Autodesk Inventor part; units mm, degrees
(part 3 of 3)
sketch "Эскиз41" plane through (1.5, 0, 0) normal (1, 0, 0) x (0, 0, -1)
  circle A0 centre (383.6, 368.9) radius 1.625 projected
  circle A1 centre (-13.6, 369) radius 1.625 projected
  circle A2 centre (383.6, 1.1) radius 1.625 projected
  circle A3 centre (-13.6, 1.1) radius 1.625 projected
  circle A4 centre (379.0468, 185.0848) radius 1.625 projected
  circle A5 centre (-9.0468, 185.0848) radius 1.625 projected
  circle A6 centre (379, 228) radius 1.625 projected
  circle A7 centre (-9, 228) radius 1.625 projected
  circle A8 centre (316, 368) radius 1.625 projected
  circle A9 centre (299, 228) radius 1.625 projected
  circle A10 centre (54, 228) radius 1.625 projected
  circle A11 centre (71, 142) radius 1.625 projected
  circle A12 centre (71, 2.0002) radius 1.625 projected
  circle A13 centre (54, 2.0002) radius 1.625 projected
  circle A14 centre (71, 368) radius 1.625 projected
  circle A15 centre (71, 228) radius 1.625 projected
  circle A16 centre (316, 142) radius 1.625 projected
  circle A17 centre (316, 228) radius 1.625 projected
  circle A18 centre (183.175, 129.0059) radius 1.85 projected
  circle A19 centre (299, 368) radius 1.625 projected
  circle A20 centre (316, 2.0002) radius 1.625 projected
  circle A21 centre (54, 142) radius 1.625 projected
  circle A22 centre (54, 368) radius 1.625 projected
  circle A23 centre (299, 2.0002) radius 1.625 projected
  circle A24 centre (299, 142) radius 1.625 projected
  arc A25 (185, 193.309) -> (185, 192.7028) centre (183.175, 193.0059) ccw projected
  line L0 (185, 193.309) -> (185, 192.7028) projected
  line L1 (14.5, 247.5001) -> (35, 247.5001) projected
  arc A26 (38, 244.5001) -> (35, 247.5001) centre (35, 244.5001) ccw projected
  line L2 (38, 244.5001) -> (38, 185.5001) projected
  arc A27 (35, 182.5001) -> (38, 185.5001) centre (35, 185.5001) ccw projected
  line L3 (35, 182.5001) -> (14.5, 182.5001) projected
  arc A28 (11.5, 185.5001) -> (14.5, 182.5001) centre (14.5, 185.5001) ccw projected
  line L4 (11.5, 185.5001) -> (11.5, 244.5001) projected
  arc A29 (14.5, 247.5001) -> (11.5, 244.5001) centre (14.5, 244.5001) ccw projected
  line L5 (358.5, 244.5001) -> (358.5, 185.5001) projected
  arc A30 (355.5, 182.5001) -> (358.5, 185.5001) centre (355.5, 185.5001) ccw projected
  line L6 (355.5, 182.5001) -> (335, 182.5001) projected
  arc A31 (332, 185.5001) -> (335, 182.5001) centre (335, 185.5001) ccw projected
  line L7 (332, 185.5001) -> (332, 244.5001) projected
  arc A32 (335, 247.5001) -> (332, 244.5001) centre (335, 244.5001) ccw projected
  line L8 (335, 247.5001) -> (355.5, 247.5001) projected
  arc A33 (358.5, 244.5001) -> (355.5, 247.5001) centre (355.5, 244.5001) ccw projected
  line L9 (98.825, 226.3849) -> (98.825, 137.3849) projected
  arc A34 (95.825, 134.3849) -> (98.825, 137.3849) centre (95.825, 137.3849) ccw projected
  line L10 (95.825, 134.3849) -> (87.825, 134.3849) projected
  arc A35 (84.825, 137.3849) -> (87.825, 134.3849) centre (87.825, 137.3849) ccw projected
  line L11 (84.825, 137.3849) -> (84.825, 226.3849) projected
  arc A36 (87.825, 229.3849) -> (84.825, 226.3849) centre (87.825, 226.3849) ccw projected
  line L12 (87.825, 229.3849) -> (95.825, 229.3849) projected
  arc A37 (98.825, 226.3849) -> (95.825, 229.3849) centre (95.825, 226.3849) ccw projected
  circle A38 centre (124.375, 129.0059) radius 2 projected
  circle A39 centre (124.375, 193.0059) radius 2 projected
  circle A40 centre (217.25, 312.9941) radius 2.1 projected
  circle A41 centre (152.75, 57.0059) radius 2.1 projected
  circle A42 centre (152.75, 118.0059) radius 2.1 projected
  circle A43 centre (152.75, 312.9941) radius 2.1 projected
  circle A44 centre (217.25, 251.9941) radius 2.1 projected
  circle A45 centre (217.25, 57.0059) radius 2.1 projected
  circle A46 centre (217.25, 118.0059) radius 2.1 projected
  circle A47 centre (152.75, 251.9941) radius 2.1 projected
  line L13 (165, 44) -> (165, 8) projected
  arc A48 (162, 5) -> (165, 8) centre (162, 8) ccw projected
  line L14 (162, 5) -> (96, 5) projected
  arc A49 (93, 8) -> (96, 5) centre (96, 8) ccw projected
  line L15 (93, 8) -> (93, 44) projected
  arc A50 (96, 47) -> (93, 44) centre (96, 44) ccw projected
  line L16 (96, 47) -> (162, 47) projected
  arc A51 (165, 44) -> (162, 47) centre (162, 44) ccw projected
  circle A52 centre (319.1128, 165.0002) radius 2.1 projected
  circle A53 centre (287, 56.343) radius 2.1 projected
  circle A54 centre (50.8872, 165.0002) radius 2.1 projected
  circle A55 centre (173.9908, 56.343) radius 2.1 projected
  circle A56 centre (135.25, 60) radius 2.1 projected
  circle A57 centre (103, 60) radius 2.1 projected
  line L17 (226.25, 270.0041) -> (226.25, 298.657) projected
  arc A58 (228.25, 300.657) -> (226.25, 298.657) centre (228.25, 298.657) ccw projected
  line L18 (228.25, 300.657) -> (268.3252, 300.657) projected
  arc A59 (269.4885, 297.03) -> (268.3252, 300.657) centre (268.3252, 298.657) ccw projected
  line L19 (269.4885, 297.03) -> (229.4132, 268.3772) projected
  arc A60 (226.25, 270.0041) -> (229.4132, 268.3772) centre (228.25, 270.0041) ccw projected
  arc A61 (235.9248, 170.343) -> (234.7615, 166.7161) centre (235.9248, 168.343) ccw projected
  line L20 (235.9248, 170.343) -> (276, 170.343) projected
  arc A62 (278, 168.343) -> (276, 170.343) centre (276, 168.343) ccw projected
  line L21 (278, 168.343) -> (278, 139.6902) projected
  arc A63 (274.8368, 138.0633) -> (278, 139.6902) centre (276, 139.6902) ccw projected
  line L22 (274.8368, 138.0633) -> (234.7615, 166.7161) projected
  arc A64 (94, 106.343) -> (92, 104.343) centre (94, 104.343) ccw projected
  line L23 (94, 106.343) -> (134.0752, 106.343) projected
  arc A65 (135.2385, 102.7161) -> (134.0752, 106.343) centre (134.0752, 104.343) ccw projected
  line L24 (135.2385, 102.7161) -> (95.1632, 74.0633) projected
  arc A66 (92, 75.6902) -> (95.1632, 74.0633) centre (94, 75.6902) ccw projected
  line L25 (92, 75.6902) -> (92, 104.343) projected
  arc A67 (92, 265.657) -> (94, 263.657) centre (94, 265.657) ccw projected
  line L26 (92, 265.657) -> (92, 294.3098) projected
  arc A68 (95.1632, 295.9367) -> (92, 294.3098) centre (94, 294.3098) ccw projected
  line L27 (95.1632, 295.9367) -> (135.2385, 267.2839) projected
  arc A69 (134.0752, 263.657) -> (135.2385, 267.2839) centre (134.0752, 265.657) ccw projected
  line L28 (134.0752, 263.657) -> (94, 263.657) projected
  arc A70 (130.725, 206.0059) -> (132.725, 204.0059) centre (132.725, 206.0059) ccw projected
  line L29 (130.725, 206.0059) -> (130.725, 234.2716) projected
  arc A71 (133.9769, 235.8314) -> (130.725, 234.2716) centre (132.725, 234.2716) ccw projected
  line L30 (133.9769, 235.8314) -> (169.1945, 207.5656) projected
  arc A72 (167.9426, 204.0059) -> (169.1945, 207.5656) centre (167.9426, 206.0059) ccw projected
  line L31 (167.9426, 204.0059) -> (132.725, 204.0059) projected
  arc A73 (226.25, 71.343) -> (228.25, 69.343) centre (228.25, 71.343) ccw projected
  line L32 (226.25, 71.343) -> (226.25, 99.9959) projected
  arc A74 (229.4132, 101.6228) -> (226.25, 99.9959) centre (228.25, 99.9959) ccw projected
  line L33 (229.4132, 101.6228) -> (269.4885, 72.97) projected
  arc A75 (268.3252, 69.343) -> (269.4885, 72.97) centre (268.3252, 71.343) ccw projected
  line L34 (268.3252, 69.343) -> (228.25, 69.343) projected
  arc A76 (226.25, 201.657) -> (228.25, 199.657) centre (228.25, 201.657) ccw projected
  line L35 (226.25, 201.657) -> (226.25, 230.3098) projected
  arc A77 (229.4132, 231.9367) -> (226.25, 230.3098) centre (228.25, 230.3098) ccw projected
  line L36 (229.4132, 231.9367) -> (269.4885, 203.2839) projected
  arc A78 (268.3252, 199.657) -> (269.4885, 203.2839) centre (268.3252, 201.657) ccw projected
  line L37 (268.3252, 199.657) -> (228.25, 199.657) projected
  arc A79 (278, 294.3098) -> (274.8368, 295.9367) centre (276, 294.3098) ccw projected
  line L38 (278, 294.3098) -> (278, 265.657) projected
  arc A80 (276, 263.657) -> (278, 265.657) centre (276, 265.657) ccw projected
  line L39 (276, 263.657) -> (235.9248, 263.657) projected
  arc A81 (234.7615, 267.2839) -> (235.9248, 263.657) centre (235.9248, 265.657) ccw projected
  line L40 (234.7615, 267.2839) -> (274.8368, 295.9367) projected
  arc A82 (226.25, 135.343) -> (228.25, 133.343) centre (228.25, 135.343) ccw projected
  line L41 (226.25, 135.343) -> (226.25, 163.9959) projected
  arc A83 (229.4132, 165.6228) -> (226.25, 163.9959) centre (228.25, 163.9959) ccw projected
  line L42 (229.4132, 165.6228) -> (269.4885, 136.97) projected
  arc A84 (268.3252, 133.343) -> (269.4885, 136.97) centre (268.3252, 135.343) ccw projected
  line L43 (268.3252, 133.343) -> (228.25, 133.343) projected
  arc A85 (143.75, 99.9959) -> (140.5868, 101.6228) centre (141.75, 99.9959) ccw projected
  line L44 (143.75, 99.9959) -> (143.75, 71.343) projected
  arc A86 (141.75, 69.343) -> (143.75, 71.343) centre (141.75, 71.343) ccw projected
  line L45 (141.75, 69.343) -> (101.6748, 69.343) projected
  arc A87 (100.5115, 72.97) -> (101.6748, 69.343) centre (101.6748, 71.343) ccw projected
  line L46 (100.5115, 72.97) -> (140.5868, 101.6228) projected
  arc A88 (143.75, 298.657) -> (141.75, 300.657) centre (141.75, 298.657) ccw projected
  line L47 (143.75, 298.657) -> (143.75, 270.0041) projected
  arc A89 (140.5868, 268.3772) -> (143.75, 270.0041) centre (141.75, 270.0041) ccw projected
  line L48 (140.5868, 268.3772) -> (100.5115, 297.03) projected
  arc A90 (101.6748, 300.657) -> (100.5115, 297.03) centre (101.6748, 298.657) ccw projected
  line L49 (101.6748, 300.657) -> (141.75, 300.657) projected
  line L50 (176.825, 239.0059) -> (176.825, 210.7401) projected
  arc A91 (173.5731, 209.1803) -> (176.825, 210.7401) centre (174.825, 210.7401) ccw projected
  line L51 (173.5731, 209.1803) -> (138.3555, 237.4461) projected
  arc A92 (139.6074, 241.0059) -> (138.3555, 237.4461) centre (139.6074, 239.0059) ccw projected
  line L52 (139.6074, 241.0059) -> (174.825, 241.0059) projected
  arc A93 (176.825, 239.0059) -> (174.825, 241.0059) centre (174.825, 239.0059) ccw projected
  line L53 (278, 104.343) -> (278, 75.6902) projected
  arc A94 (274.8368, 74.0633) -> (278, 75.6902) centre (276, 75.6902) ccw projected
  line L54 (274.8368, 74.0633) -> (234.7615, 102.7161) projected
  arc A95 (235.9248, 106.343) -> (234.7615, 102.7161) centre (235.9248, 104.343) ccw projected
  line L55 (235.9248, 106.343) -> (276, 106.343) projected
  arc A96 (278, 104.343) -> (276, 106.343) centre (276, 104.343) ccw projected
  arc A97 (278, 234.657) -> (276, 236.657) centre (276, 234.657) ccw projected
  line L56 (278, 234.657) -> (278, 206.0041) projected
  arc A98 (274.8368, 204.3772) -> (278, 206.0041) centre (276, 206.0041) ccw projected
  line L57 (274.8368, 204.3772) -> (234.7615, 233.03) projected
  arc A99 (235.9248, 236.657) -> (234.7615, 233.03) centre (235.9248, 234.657) ccw projected
  line L58 (235.9248, 236.657) -> (276, 236.657) projected
  arc A100 (295, 375) -> (292, 372) centre (295, 372) ccw projected
  line L59 (292, 372) -> (292, 323.5966) projected
  arc A101 (289, 320.5966) -> (292, 323.5966) centre (289, 323.5966) ccw projected
  line L60 (289, 320.5966) -> (81, 320.5966) projected
  arc A102 (78, 323.5966) -> (81, 320.5966) centre (81, 323.5966) ccw projected
  line L61 (78, 323.5966) -> (78, 372) projected
  arc A103 (78, 372) -> (75, 375) centre (75, 372) ccw projected
  line L62 (75, 375) -> (-15, 375) projected
  arc A104 (-15, 375) -> (-18, 372) centre (-15, 372) ccw projected
  line L63 (-18, 372) -> (-18, -2) projected
  arc A105 (-18, -2) -> (-15, -5) centre (-15, -2) ccw projected
  line L64 (-15, -5) -> (385, -5) projected
  arc A106 (385, -5) -> (388, -2) centre (385, -2) ccw projected
  line L65 (388, -2) -> (388, 372) projected
  arc A107 (388, 372) -> (385, 375) centre (385, 372) ccw projected
  line L66 (385, 375) -> (295, 375) projected
  line L67 (49, 266.848) -> (-8, 266.848) projected
  arc A108 (-11, 269.848) -> (-8, 266.848) centre (-8, 269.848) ccw projected
  line L68 (-11, 269.848) -> (-11, 367) projected
  arc A109 (-8, 370) -> (-11, 367) centre (-8, 367) ccw projected
  line L69 (-8, 370) -> (-7.7889, 370) projected
  arc A110 (-4.2111, 370) -> (-7.7889, 370) centre (-6, 368.9) ccw projected
  line L70 (-4.2111, 370) -> (37, 370) projected
  arc A111 (40, 367) -> (37, 370) centre (37, 367) ccw projected
  line L71 (40, 367) -> (40, 341.848) projected
  arc A112 (40, 341.848) -> (43, 338.848) centre (43, 341.848) ccw projected
  line L72 (43, 338.848) -> (49, 338.848) projected
  arc A113 (52, 335.848) -> (49, 338.848) centre (49, 335.848) ccw projected
  line L73 (52, 335.848) -> (52, 269.848) projected
  arc A114 (49, 266.848) -> (52, 269.848) centre (49, 269.848) ccw projected
  line L74 (374.2111, 0) -> (333, 0) projected
  arc A115 (330, 3) -> (333, 0) centre (333, 3) ccw projected
  line L75 (330, 3) -> (330, 28.152) projected
  arc A116 (330, 28.152) -> (327, 31.152) centre (327, 28.152) ccw projected
  line L76 (327, 31.152) -> (321, 31.152) projected
  arc A117 (318, 34.152) -> (321, 31.152) centre (321, 34.152) ccw projected
  line L77 (318, 34.152) -> (318, 100.152) projected
  arc A118 (321, 103.152) -> (318, 100.152) centre (321, 100.152) ccw projected
  line L78 (321, 103.152) -> (327, 103.152) projected
  arc A119 (327, 103.152) -> (330, 106.152) centre (327, 106.152) ccw projected
  line L79 (330, 106.152) -> (330, 160) projected
  arc A120 (333, 163) -> (330, 160) centre (333, 160) ccw projected
  line L80 (333, 163) -> (377, 163) projected
  arc A121 (380, 160) -> (377, 163) centre (377, 160) ccw projected
  line L81 (380, 160) -> (380, 3) projected
  arc A122 (377.8605, 0.1261) -> (380, 3) centre (377, 3) ccw projected
  arc A123 (374.2111, 0) -> (377.8605, 0.1261) centre (376, 1.1) ccw projected
  line L82 (-7, 163) -> (37, 163) projected
  arc A124 (40, 160) -> (37, 163) centre (37, 160) ccw projected
  line L83 (40, 160) -> (40, 106.152) projected
  arc A125 (40, 106.152) -> (43, 103.152) centre (43, 106.152) ccw projected
  line L84 (43, 103.152) -> (49, 103.152) projected
  arc A126 (52, 100.152) -> (49, 103.152) centre (49, 100.152) ccw projected
  line L85 (52, 100.152) -> (52, 34.152) projected
  arc A127 (49, 31.152) -> (52, 34.152) centre (49, 34.152) ccw projected
  line L86 (49, 31.152) -> (43, 31.152) projected
  arc A128 (43, 31.152) -> (40, 28.152) centre (43, 28.152) ccw projected
  line L87 (40, 28.152) -> (40, 3) projected
  arc A129 (37, 0) -> (40, 3) centre (37, 3) ccw projected
  line L88 (37, 0) -> (-4.2111, 0) projected
  arc A130 (-7.8605, 0.1261) -> (-4.2111, 0) centre (-6, 1.1) ccw projected
  arc A131 (-10, 3) -> (-7.8605, 0.1261) centre (-7, 3) ccw projected
  line L89 (-10, 3) -> (-10, 160) projected
  arc A132 (-7, 163) -> (-10, 160) centre (-7, 160) ccw projected
  line L90 (377, 266.848) -> (321, 266.848) projected
  arc A133 (318, 269.848) -> (321, 266.848) centre (321, 269.848) ccw projected
  line L91 (318, 269.848) -> (318, 335.848) projected
  arc A134 (321, 338.848) -> (318, 335.848) centre (321, 335.848) ccw projected
  line L92 (321, 338.848) -> (327, 338.848) projected
  arc A135 (327, 338.848) -> (330, 341.848) centre (327, 341.848) ccw projected
  line L93 (330, 341.848) -> (330, 367) projected
  arc A136 (333, 370) -> (330, 367) centre (333, 367) ccw projected
  line L94 (333, 370) -> (374.2111, 370) projected
  arc A137 (377.8605, 369.8739) -> (374.2111, 370) centre (376, 368.9) ccw projected
  arc A138 (380, 367) -> (377.8605, 369.8739) centre (377, 367) ccw projected
  line L95 (380, 367) -> (380, 269.848) projected
  arc A139 (377, 266.848) -> (380, 269.848) centre (377, 269.848) ccw projected
  circle A140 centre (-7, 3) radius 3
  line L96 (-4.2111, 0) -> (-7, 0)
  circle A141 centre (377, 3) radius 3
  line L97 (374.2111, 0) -> (377, 0)
  line L98 (-18, -2) -> (-18, 372) projected
  circle A142 centre (-7, 367) radius 3
  line L99 (-4.2111, 370) -> (-7, 370)
  circle A143 centre (377, 367) radius 3
  line L100 (374.2111, 370) -> (377, 370)
  line L101 (185, -5) -> (185, 9)
  line L102 (-7, 266.848) -> (49, 266.848)
  arc A144 (49, 266.848) -> (52, 269.848) centre (49, 269.848) ccw
  line L103 (52, 269.848) -> (52, 335.848)
  arc A145 (52, 335.848) -> (49, 338.848) centre (49, 335.848) ccw
  line L104 (49, 338.848) -> (43, 338.848)
  arc A146 (40, 341.848) -> (43, 338.848) centre (43, 341.848) ccw
  line L105 (40, 341.848) -> (40, 367)
  arc A147 (40, 367) -> (37, 370) centre (37, 367) ccw
  line L106 (37, 370) -> (-4.2111, 370)
  line L107 (-10, 367) -> (-10, 269.848)
  arc A148 (-10, 269.848) -> (-7, 266.848) centre (-7, 269.848) ccw
  circle A149 centre (-7, 367) radius 3
  line L108 (-4.2111, 370) -> (-7, 370)
  point P0 (0, 0)
  point P1 (377.8605, 0.1261)
  constraints: 24 end point, 10 point on circle, 9 symmetric about line, 5 centre point, 2 coincident, 2 vertical, 1 horizontal, 1 midpoint, 1 vertical alignment, 20 other
extrude "Выдавливание35" add sketch "Эскиз41" against normal blind 1.5 contours L67 A108 L68 A109 L69 A110 L99 A142 L107 A148 | L97 A141 A123 | A140 L96 A130 | A143 L100 A137
equation "\"d99\" = d97"
